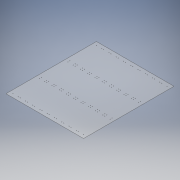
# Autodesk Inventor part: PRT1001-213 Base
Saved by Autodesk Inventor 2019 (Build 230136000, 136)
## iProperties
Created: 2019-07-02
Part Number: PRT1001-213 Base
Material: Generic
Document SubType Name: Modeling
Designer: james
Density: 1 g/cm^3
Appearance: Polycarbonate - Clear
Author: james
Autodesk Inventor part; units mm, degrees
ref_plane "YZ Plane" through (0, 0, 0) normal (1, 0, 0) x (0, 1, 0)
ref_plane "XZ Plane" through (0, 0, 0) normal (0, 1, 0) x (-1, 0, 0)
ref_plane "XY Plane" through (0, 0, 0) normal (0, 0, 1) x (1, 0, 0)
sketch "Sketch3" plane through (0, 0, 0) normal (0, 1, 0) x (-1, 0, 0)
  line L0 (447.8905, 299.355) -> (-108.1095, 299.355)
  line L1 (-108.1095, 299.355) -> (-108.1095, -348.645)
  line L2 (-108.1095, -348.645) -> (447.8905, -348.645)
  line L3 (447.8905, -348.645) -> (447.8905, 299.355)
  point P0 (0, 0)
  dimension "d19" = 648
  dimension "d20" = 556
  constraints: 8 end point, 2 parallel, 1 horizontal, 1 perpendicular
  measures "d19" distance of L0.end L1.end
  measures "d20" distance of L0.start L0.end
extrude "Extrusion2" add sketch "Sketch3" along normal blind 1
sketch "Sketch4" plane through (0, 1, 0) normal (0, 1, 0) x (1, 0, 0)
  line L0 (108.1095, 348.645) -> (-447.8905, 348.645) projected
  line L1 (108.1095, -299.355) -> (108.1095, 348.645) projected
  point P0 (0, 0)
  point P1 (83.1095, 323.645)
  point P2 (45.1095, 323.645)
  point P3 (45.1095, 133.645)
  point P4 (83.1095, 133.645)
  point P5 (83.1095, 119.645)
  point P6 (45.1095, 119.645)
  point P7 (45.1095, -70.355)
  point P8 (83.1095, -70.355)
  point P9 (83.1095, -84.355)
  point P10 (45.1095, -84.355)
  point P11 (45.1095, -274.355)
  point P12 (83.1095, -274.355)
  point P13 (31.1095, 323.645)
  point P14 (-6.8905, 323.645)
  point P15 (-6.8905, 133.645)
  point P16 (31.1095, 133.645)
  point P17 (31.1095, -70.355)
  point P18 (-6.8905, -70.355)
  point P19 (-6.8905, 119.645)
  point P20 (31.1095, 119.645)
  point P21 (31.1095, -274.355)
  point P22 (-6.8905, -274.355)
  point P23 (-6.8905, -84.355)
  point P24 (31.1095, -84.355)
  point P25 (-20.8905, 323.645)
  point P26 (-58.8905, 323.645)
  point P27 (-58.8905, 133.645)
  point P28 (-20.8905, 133.645)
  point P29 (-20.8905, -70.355)
  point P30 (-58.8905, -70.355)
  point P31 (-58.8905, 119.645)
  point P32 (-20.8905, 119.645)
  point P33 (-20.8905, -274.355)
  point P34 (-58.8905, -274.355)
  point P35 (-58.8905, -84.355)
  point P36 (-20.8905, -84.355)
  point P37 (-72.8905, -84.355)
  point P38 (-110.8905, -84.355)
  point P39 (-110.8905, -274.355)
  point P40 (-72.8905, -274.355)
  point P41 (-72.8905, 119.645)
  point P42 (-110.8905, 119.645)
  point P43 (-110.8905, -70.355)
  point P44 (-72.8905, -70.355)
  point P45 (-72.8905, 133.645)
  point P46 (-110.8905, 133.645)
  point P47 (-110.8905, 323.645)
  point P48 (-72.8905, 323.645)
  point P49 (-124.8905, 323.645)
  point P50 (-162.8905, 323.645)
  point P51 (-162.8905, 133.645)
  point P52 (-124.8905, 133.645)
  point P53 (-124.8905, -70.355)
  point P54 (-162.8905, -70.355)
  point P55 (-162.8905, 119.645)
  point P56 (-124.8905, 119.645)
  point P57 (-124.8905, -274.355)
  point P58 (-162.8905, -274.355)
  point P59 (-162.8905, -84.355)
  point P60 (-124.8905, -84.355)
  point P61 (-176.8905, -84.355)
  point P62 (-214.8905, -84.355)
  point P63 (-214.8905, -274.355)
  point P64 (-176.8905, -274.355)
  point P65 (-176.8905, 119.645)
  point P66 (-214.8905, 119.645)
  point P67 (-214.8905, -70.355)
  point P68 (-176.8905, -70.355)
  point P69 (-176.8905, 133.645)
  point P70 (-214.8905, 133.645)
  point P71 (-214.8905, 323.645)
  point P72 (-176.8905, 323.645)
  point P73 (-280.8905, 323.645)
  point P74 (-318.8905, 323.645)
  point P75 (-318.8905, 133.645)
  point P76 (-280.8905, 133.645)
  point P77 (-280.8905, -70.355)
  point P78 (-318.8905, -70.355)
  point P79 (-318.8905, 119.645)
  point P80 (-280.8905, 119.645)
  point P81 (-280.8905, -274.355)
  point P82 (-318.8905, -274.355)
  point P83 (-318.8905, -84.355)
  point P84 (-280.8905, -84.355)
  point P85 (-228.8905, -84.355)
  point P86 (-266.8905, -84.355)
  point P87 (-266.8905, -274.355)
  point P88 (-228.8905, -274.355)
  point P89 (-228.8905, 119.645)
  point P90 (-266.8905, 119.645)
  point P91 (-266.8905, -70.355)
  point P92 (-228.8905, -70.355)
  point P93 (-228.8905, 133.645)
  point P94 (-266.8905, 133.645)
  point P95 (-266.8905, 323.645)
  point P96 (-228.8905, 323.645)
  point P97 (-332.8905, 323.645)
  point P98 (-370.8905, 323.645)
  point P99 (-370.8905, 133.645)
  point P100 (-332.8905, 133.645)
  point P101 (-332.8905, -70.355)
  point P102 (-370.8905, -70.355)
  point P103 (-370.8905, 119.645)
  point P104 (-332.8905, 119.645)
  point P105 (-332.8905, -274.355)
  point P106 (-370.8905, -274.355)
  point P107 (-370.8905, -84.355)
  point P108 (-332.8905, -84.355)
  point P109 (-384.8905, -84.355)
  point P110 (-422.8905, -84.355)
  point P111 (-422.8905, -274.355)
  point P112 (-384.8905, -274.355)
  point P113 (-384.8905, 119.645)
  point P114 (-422.8905, 119.645)
  point P115 (-422.8905, -70.355)
  point P116 (-384.8905, -70.355)
  point P117 (-384.8905, 133.645)
  point P118 (-422.8905, 133.645)
  point P119 (-422.8905, 323.645)
  point P120 (-384.8905, 323.645)
  dimension "d23" = 25
  dimension "d24" = 25
  dimension "d34" = 0
  dimension "d35" = 0
  dimension "d36" = 0
  dimension "d37" = 0
  dimension "d38" = 190
  dimension "d39" = 38
  dimension "d40" = 0
  dimension "d41" = 0
  dimension "d42" = 0
  dimension "d43" = 0
  dimension "d44" = 190
  dimension "d45" = 38
  dimension "d48" = 0
  dimension "d49" = 0
  dimension "d50" = 0
  dimension "d51" = 0
  dimension "d52" = 190
  dimension "d53" = 38
  dimension "d56" = 0
  dimension "d57" = 14
  dimension "d58" = 0
  dimension "d59" = 14
  dimension "d60" = 0
  dimension "d61" = 0
  dimension "d62" = 0
  dimension "d63" = 0
  dimension "d64" = 190
  dimension "d65" = 38
  dimension "d66" = 0
  dimension "d67" = 0
  dimension "d68" = 0
  dimension "d69" = 0
  dimension "d70" = 190
  dimension "d71" = 38
  dimension "d72" = 0
  dimension "d73" = 0
  dimension "d74" = 0
  dimension "d75" = 0
  dimension "d76" = 190
  dimension "d77" = 38
  dimension "d78" = 0
  dimension "d79" = 14
  dimension "d80" = 0
  dimension "d81" = 14
  dimension "d89" = 0
  dimension "d90" = 14
  dimension "d91" = 0
  dimension "d92" = 0
  dimension "d93" = 0
  dimension "d94" = 0
  dimension "d95" = 190
  dimension "d96" = 38
  dimension "d97" = 0
  dimension "d98" = 0
  dimension "d99" = 0
  dimension "d100" = 0
  dimension "d101" = 190
  dimension "d102" = 38
  dimension "d103" = 0
  dimension "d104" = 0
  dimension "d105" = 0
  dimension "d106" = 0
  measures "d23" distance from line of L0 point (83.11, 323.645)
  measures "d24" distance from line of L1 point (83.11, 323.645)
  measures "d34" horizontal distance of point (83.11, 133.645) point (83.11, 323.645)
  measures "d35" horizontal distance of point (45.11, 323.645) point (45.11, 133.645)
  measures "d36" vertical distance of point (83.11, 323.645) point (45.11, 323.645)
  measures "d37" vertical distance of point (83.11, 133.645) point (45.11, 133.645)
  measures "d38" distance of point (83.11, 323.645) point (83.11, 133.645)
  measures "d39" distance of point (83.11, 323.645) point (45.11, 323.645)
  measures "d40" horizontal distance of point (83.11, -70.355) point (83.11, 119.645)
  measures "d41" horizontal distance of point (45.11, 119.645) point (45.11, -70.355)
  measures "d42" vertical distance of point (83.11, 119.645) point (45.11, 119.645)
  measures "d43" vertical distance of point (83.11, -70.355) point (45.11, -70.355)
  measures "d44" distance of point (83.11, 119.645) point (83.11, -70.355)
  measures "d45" distance of point (83.11, 119.645) point (45.11, 119.645)
  measures "d48" horizontal distance of point (83.11, -274.355) point (83.11, -84.355)
  measures "d49" horizontal distance of point (45.11, -84.355) point (45.11, -274.355)
  measures "d50" vertical distance of point (83.11, -84.355) point (45.11, -84.355)
  measures "d51" vertical distance of point (83.11, -274.355) point (45.11, -274.355)
  measures "d52" distance of point (83.11, -84.355) point (83.11, -274.355)
  measures "d53" distance of point (83.11, -84.355) point (45.11, -84.355)
  measures "d56" horizontal distance of point (83.11, 133.645) point (83.11, 119.645)
  measures "d57" distance of point (83.11, 133.645) point (83.11, 119.645)
  measures "d58" horizontal distance of point (83.11, -84.355) point (83.11, -70.355)
  measures "d59" distance of point (83.11, -70.355) point (83.11, -84.355)
  measures "d60" horizontal distance of point (31.11, 133.645) point (31.11, 323.645)
  measures "d61" horizontal distance of point (-6.89, 323.645) point (-6.89, 133.645)
  measures "d62" vertical distance of point (31.11, 323.645) point (-6.89, 323.645)
  measures "d63" vertical distance of point (31.11, 133.645) point (-6.89, 133.645)
  measures "d64" distance of point (31.11, 323.645) point (31.11, 133.645)
  measures "d65" distance of point (31.11, 323.645) point (-6.89, 323.645)
  measures "d66" horizontal distance of point (31.11, -70.355) point (31.11, 119.645)
  measures "d67" horizontal distance of point (-6.89, 119.645) point (-6.89, -70.355)
  measures "d68" vertical distance of point (31.11, 119.645) point (-6.89, 119.645)
  measures "d69" vertical distance of point (31.11, -70.355) point (-6.89, -70.355)
  measures "d70" distance of point (31.11, 119.645) point (31.11, -70.355)
  measures "d71" distance of point (31.11, 119.645) point (-6.89, 119.645)
  measures "d72" horizontal distance of point (31.11, -274.355) point (31.11, -84.355)
  measures "d73" horizontal distance of point (-6.89, -84.355) point (-6.89, -274.355)
  measures "d74" vertical distance of point (31.11, -84.355) point (-6.89, -84.355)
  measures "d75" vertical distance of point (31.11, -274.355) point (-6.89, -274.355)
  measures "d76" distance of point (31.11, -84.355) point (31.11, -274.355)
  measures "d77" distance of point (31.11, -84.355) point (-6.89, -84.355)
  measures "d78" horizontal distance of point (31.11, 133.645) point (31.11, 119.645)
  measures "d79" distance of point (31.11, 133.645) point (31.11, 119.645)
  measures "d80" horizontal distance of point (31.11, -84.355) point (31.11, -70.355)
  measures "d81" distance of point (31.11, -70.355) point (31.11, -84.355)
  measures "d89" vertical distance of point (45.11, -274.355) point (31.11, -274.355)
  measures "d90" distance of point (45.11, -274.355) point (31.11, -274.355)
  measures "d91" horizontal distance of point (-20.89, 133.645) point (-20.89, 323.645)
  measures "d92" horizontal distance of point (-58.89, 323.645) point (-58.89, 133.645)
  measures "d93" vertical distance of point (-20.89, 323.645) point (-58.89, 323.645)
  measures "d94" vertical distance of point (-20.89, 133.645) point (-58.89, 133.645)
  measures "d95" distance of point (-20.89, 323.645) point (-20.89, 133.645)
  measures "d96" distance of point (-20.89, 323.645) point (-58.89, 323.645)
  measures "d97" horizontal distance of point (-20.89, -70.355) point (-20.89, 119.645)
  measures "d98" horizontal distance of point (-58.89, 119.645) point (-58.89, -70.355)
  measures "d99" vertical distance of point (-20.89, 119.645) point (-58.89, 119.645)
  measures "d100" vertical distance of point (-20.89, -70.355) point (-58.89, -70.355)
  measures "d101" distance of point (-20.89, 119.645) point (-20.89, -70.355)
  measures "d102" distance of point (-20.89, 119.645) point (-58.89, 119.645)
  measures "d103" horizontal distance of point (-20.89, -274.355) point (-20.89, -84.355)
  measures "d104" horizontal distance of point (-58.89, -84.355) point (-58.89, -274.355)
  measures "d105" vertical distance of point (-20.89, -84.355) point (-58.89, -84.355)
  measures "d106" vertical distance of point (-20.89, -274.355) point (-58.89, -274.355)
hole "Hole3" at (83.1095, 1, -323.645) at (45.1095, 1, -323.645) at (45.1095, 1, -133.645) at (83.1095, 1, -133.645) at (83.1095, 1, 70.355) at (45.1095, 1, 70.355) at (45.1095, 1, -119.645) at (83.1095, 1, -119.645) at (83.1095, 1, 274.355) at (45.1095, 1, 274.355) at (45.1095, 1, 84.355) at (83.1095, 1, 84.355) at (31.1095, 1, 84.355) at (-6.8905, 1, 84.355) at (-6.8905, 1, 274.355) at (31.1095, 1, 274.355) at (31.1095, 1, -119.645) at (-6.8905, 1, -119.645) at (-6.8905, 1, 70.355) at (31.1095, 1, 70.355) at (31.1095, 1, -133.645) at (-6.8905, 1, -133.645) at (-6.8905, 1, -323.645) at (31.1095, 1, -323.645) at (-72.8905, 1, -323.645) at (-110.8905, 1, -323.645) at (-110.8905, 1, -133.645) at (-72.8905, 1, -133.645) at (-72.8905, 1, 70.355) at (-110.8905, 1, 70.355) at (-110.8905, 1, -119.645) at (-72.8905, 1, -119.645) at (-72.8905, 1, 274.355) at (-110.8905, 1, 274.355) at (-110.8905, 1, 84.355) at (-72.8905, 1, 84.355) at (-20.8905, 1, 84.355) at (-58.8905, 1, 84.355) at (-58.8905, 1, 274.355) at (-20.8905, 1, 274.355) at (-20.8905, 1, -119.645) at (-58.8905, 1, -119.645) at (-58.8905, 1, 70.355) at (-20.8905, 1, 70.355) at (-20.8905, 1, -133.645) at (-58.8905, 1, -133.645) at (-58.8905, 1, -323.645) at (-20.8905, 1, -323.645) at (-228.8905, 1, -323.645) at (-266.8905, 1, -323.645) direction (0, -1, 0) diameter 3 depth 25.4 tip angle 118.188 and at (-266.8905, 1, -133.645) (-228.8905, 1, -133.645) (-228.8905, 1, 70.355) (-266.8905, 1, 70.355) (-266.8905, 1, -119.645) (-228.8905, 1, -119.645) (-228.8905, 1, 274.355) (-266.8905, 1, 274.355) (-266.8905, 1, 84.355) (-228.8905, 1, 84.355) (-280.8905, 1, 84.355) (-318.8905, 1, 84.355) (-318.8905, 1, 274.355) (-280.8905, 1, 274.355) (-280.8905, 1, -119.645) (-318.8905, 1, -119.645) (-318.8905, 1, 70.355) (-280.8905, 1, 70.355) (-280.8905, 1, -133.645) (-318.8905, 1, -133.645) (-318.8905, 1, -323.645) (-280.8905, 1, -323.645) (-176.8905, 1, -323.645) (-214.8905, 1, -323.645) (-214.8905, 1, -133.645) (-176.8905, 1, -133.645) (-176.8905, 1, 70.355) (-214.8905, 1, 70.355) (-214.8905, 1, -119.645) (-176.8905, 1, -119.645) (-176.8905, 1, 274.355) (-214.8905, 1, 274.355) (-214.8905, 1, 84.355) (-176.8905, 1, 84.355) (-124.8905, 1, 84.355) (-162.8905, 1, 84.355) (-162.8905, 1, 274.355) (-124.8905, 1, 274.355) (-124.8905, 1, -119.645) (-162.8905, 1, -119.645) (-162.8905, 1, 70.355) (-124.8905, 1, 70.355) (-124.8905, 1, -133.645) (-162.8905, 1, -133.645) (-162.8905, 1, -323.645) (-124.8905, 1, -323.645) (-384.8905, 1, -323.645) (-422.8905, 1, -323.645) (-422.8905, 1, -133.645) (-384.8905, 1, -133.645) (-384.8905, 1, 70.355) (-422.8905, 1, 70.355) (-422.8905, 1, -119.645) (-384.8905, 1, -119.645) (-384.8905, 1, 274.355) (-422.8905, 1, 274.355) (-422.8905, 1, 84.355) (-384.8905, 1, 84.355) (-332.8905, 1, 84.355) (-370.8905, 1, 84.355) (-370.8905, 1, 274.355) (-332.8905, 1, 274.355) (-332.8905, 1, -119.645) (-370.8905, 1, -119.645) (-370.8905, 1, 70.355) (-332.8905, 1, 70.355) (-332.8905, 1, -133.645) (-370.8905, 1, -133.645) (-370.8905, 1, -323.645) (-332.8905, 1, -323.645)
equation "\"d19\" = BaseLength"
equation "\"d20\" = BaseWidth"
equation "\"d21\" = BoardHeight"
equation "\"d23\" = BaseBoardOffset + ScrewHoleOffset"
equation "\"d24\" = BaseBoardOffset + ScrewHoleOffset"
equation "\"d38\" = VertOffsetBetweenScrews"
equation "\"d39\" = HorizOffsetBetweenScrews"
equation "\"d44\" = d46"
equation "\"d45\" = d47"
equation "\"d52\" = d54"
equation "\"d53\" = d55"
equation "\"d57\" = 2 * ScrewHoleOffset + BoardGap"
equation "\"d59\" = 2 * ScrewHoleOffset + BoardGap"
equation "\"d64\" = d82"
equation "\"d65\" = d83"
equation "\"d70\" = d84"
equation "\"d71\" = d85"
equation "\"d76\" = d86"
equation "\"d77\" = d87"
equation "\"d79\" = 2 * ScrewHoleOffset + BoardGap"
equation "\"d81\" = 2 * ScrewHoleOffset + BoardGap"
equation "\"d90\" = 2 * ScrewHoleOffset + BoardGap"
equation "\"d95\" = d137"
equation "\"d96\" = d138"
equation "\"d101\" = d139"
equation "\"d102\" = d140"
equation "\"d401\" = ScrewSize"
equation "\"BoardWidth\" = 48"
equation "\"ScrewSize\" = 3"
equation "\"ScrewHoleOffset\" = 5"
equation "\"BoardGap\" = 4"
equation "\"BoardHeight\" = 1"
equation "\"BaseWidth\" = 556"
equation "\"HorizOffsetBetweenScrews\" = 38"
equation "\"VertOffsetBetweenScrews\" = 190"
equation "\"BaseBoardOffset\" = 20"
equation "\"BaseLength\" = 648"
equation "\"d46\" = 190"
equation "\"d47\" = 38"
equation "\"d54\" = 190"
equation "\"d55\" = 38"
equation "\"d82\" = 190"
equation "\"d83\" = 38"
equation "\"d84\" = 190"
equation "\"d85\" = 38"
equation "\"d86\" = 190"
equation "\"d87\" = 38"
equation "\"d88\" = 4"
equation "\"d137\" = 190"
equation "\"d138\" = 38"
equation "\"d139\" = 190"
equation "\"d140\" = 38"
equation "\"d141\" = 190"
equation "\"d142\" = 38"
equation "\"d143\" = 4"
equation "\"d144\" = 190"
equation "\"d145\" = 38"
equation "\"d146\" = 190"
equation "\"d147\" = 38"
equation "\"d148\" = 190"
equation "\"d149\" = 38"
equation "\"d150\" = 4"
equation "\"d247\" = 190"
equation "\"d248\" = 38"
equation "\"d249\" = 190"
equation "\"d250\" = 38"
equation "\"d251\" = 190"
equation "\"d252\" = 38"
equation "\"d253\" = 4"
equation "\"d254\" = 190"
equation "\"d255\" = 38"
equation "\"d256\" = 190"
equation "\"d257\" = 38"
equation "\"d258\" = 190"
equation "\"d259\" = 38"
equation "\"d260\" = 4"
equation "\"d261\" = 190"
equation "\"d262\" = 38"
equation "\"d263\" = 190"
equation "\"d264\" = 38"
equation "\"d265\" = 190"
equation "\"d266\" = 38"
equation "\"d267\" = 4"
equation "\"d268\" = 190"
equation "\"d269\" = 38"
equation "\"d270\" = 190"
equation "\"d271\" = 38"
equation "\"d272\" = 190"
equation "\"d273\" = 38"
equation "\"d274\" = 4"
equation "\"d369\" = 190"
equation "\"d370\" = 38"
equation "\"d371\" = 190"
equation "\"d372\" = 38"
equation "\"d373\" = 190"
equation "\"d374\" = 38"
equation "\"d375\" = 4"
equation "\"d376\" = 190"
equation "\"d377\" = 38"
equation "\"d378\" = 190"
equation "\"d379\" = 38"
equation "\"d380\" = 190"
equation "\"d381\" = 38"
equation "\"d382\" = 4"
equation "\"d384\" = 38"
equation "\"d386\" = 38"
equation "\"d388\" = 38"
equation "\"d389\" = 4"
equation "\"d391\" = 38"
equation "\"d393\" = 38"
equation "\"d395\" = 38"
equation "\"d396\" = 4"
body "Solid2"
